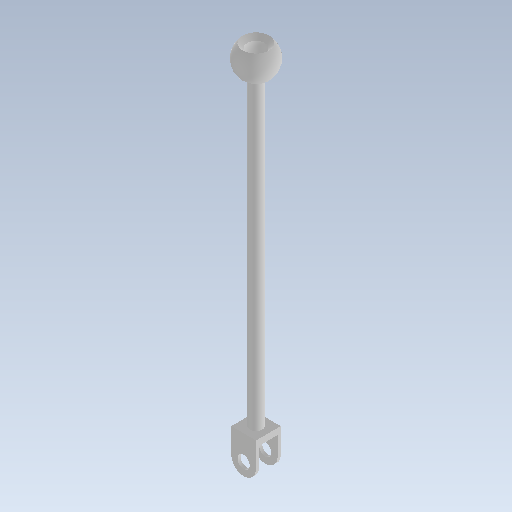
# Autodesk Inventor part: US_Dyad-01
Saved by Autodesk Inventor 2020.1 (Build 241239000, 239)
## iProperties
Created: 2019-10-24
Part Number: US_Dyad-01
Material: Generic
Document SubType Name: Modeling
Designer: sshel
Density: 1 g/cm^3
Appearance: Default
Author: sshel
Autodesk Inventor part; units mm, degrees
ref_plane "YZ Plane" through (0, 0, 0) normal (1, 0, 0) x (0, 1, 0)
ref_plane "XZ Plane" through (0, 0, 0) normal (0, 1, 0) x (-1, 0, 0)
ref_plane "XY Plane" through (0, 0, 0) normal (0, 0, 1) x (1, 0, 0)
sketch "Sketch1" plane through (0, 0, 0) normal (0, 1, 0) x (-1, 0, 0)
  line L0 (0, 0) -> (0, -5145.9)
  line L1 (-200, -4980.2146) -> (-200, 0)
  line L2 (0, 0) -> (-173.6931, 0)
  line L3 (0, 0) -> (0, 5145.9)
  line L4 (-200, 4980.2146) -> (-200, 0)
  arc A0 (-424.2641, 5970.1641) -> (-200, 4980.2146) centre (0, 5545.9) ccw
  arc A1 (-282.8427, 5828.7427) -> (0, 5145.9) centre (0, 5545.9) ccw
  line L5 (-282.8427, 5828.7427) -> (-424.2641, 5970.1641)
  line L6 (0, -7806.6864) -> (0, 8018.8184) construction
  line L7 (0, -5145.9) -> (0, -5545.9)
  line L8 (0, -5545.9) -> (-200, -5545.9)
  line L9 (-200, -5545.9) -> (-200, -4980.2146)
  point P0 (0, -2.2081)
  point P1 (-13.1062, 0)
  point P2 (-20, -18.7767)
  point P3 (-20, 3.1509)
  point P4 (-46.6023, 0)
  point P5 (-20, -18.7767)
  dimension "d6" = 45
  dimension "d7" = 200
  dimension "d8" = 400
  dimension "d9" = 200
  dimension "d10" = 11091.8
  constraints: 18 end point, 4 point on circle, 3 symmetric about line, 2 centre point, 2 horizontal, 2 point on line, 2 vertical, 1 coincident, 1 collinear, 1 perpendicular
  measures "d6" angle of L6 L5
  measures "d7" radial gap between concentric circles of A1 A0
  measures "d8" radius of A1
  measures "d9" distance between parallel lines of L4 L6
  measures "d10" distance of L7.end A1.centre
revolve "Revolution1" add sketch "Sketch1" angle 360 about axis through (0, 0, -10) along (0, 0, 1)
sketch "Sketch2" plane through (0, 0, 0) normal (0, 1, 0) x (-1, 0, 0)
  line L0 (200, -5545.9) -> (-200, -5545.9) projected
  arc A0 (-400, -5545.9) -> (400, -5545.9) centre (0, -5545.9) ccw
  line L1 (65.0556, -5545.9) -> (-85.3956, -5545.9)
  line L2 (0, -338.7665) -> (0, -580.5318)
  line L3 (400, -5545.9) -> (400, -4745.9)
  line L4 (400, -4745.9) -> (-400, -4745.9)
  line L5 (-400, -4745.9) -> (-400, -5545.9)
  point P0 (0, 0)
  dimension "d11" = 400
  dimension "d12" = 800
  constraints: 10 end point, 4 point on line, 2 perpendicular, 2 point on circle, 2 vertical, 1 centre point, 1 horizontal, 1 midpoint, 1 tangent
  measures "d11" radius of A0
  measures "d12" distance of L5.end L4.end
extrude "Extrusion1" add sketch "Sketch2" along normal mid plane 800
sketch "Sketch4" plane through (0, 0, 0) normal (0, 1, 0) x (-1, 0, 0)
  arc A0 (-400, -5545.9) -> (400, -5545.9) centre (0, -5545.9) ccw construction
  circle A1 centre (0, -5545.9) radius 200
  point P0 (0, 0)
  dimension "d16" = 200
  constraints: 1 centre point, 1 coincident
  measures "d16" radius of A1
extrude "Extrusion2" cut sketch "Sketch4" along normal through all both and the other way through all
sketch "Sketch6" plane through (0, 0, 0) normal (1, 0, 0) x (0, 1, 0)
  line L0 (-400, -5945.9) -> (400, -5945.9) construction
  line L1 (0, -623.7458) -> (0, -465.1617)
  line L2 (300, -5945.9) -> (-300, -5945.9)
  line L3 (-300, -5945.9) -> (-300, -4945.9)
  line L4 (-300, -4945.9) -> (300, -4945.9)
  line L5 (300, -4945.9) -> (300, -5945.9)
  point P0 (0, 0)
  point P1 (0, -5945.9)
  dimension "d27" = 600
  dimension "d28" = 1000
  constraints: 10 end point, 2 parallel, 1 collinear, 1 horizontal, 1 midpoint, 1 perpendicular, 1 point on line, 1 vertical, 1 other
  measures "d27" distance between parallel lines of L3 L5
  measures "d28" distance of L2.end L3.end
extrude "Extrusion4" cut sketch "Sketch6" along normal through all both and the other way through all
equation "\"d7\" = rod_radius"
equation "\"d8\" = S_radius"
equation "\"d9\" = rod_radius"
equation "\"d10\" = L1"
equation "\"d11\" = S_radius"
equation "\"d12\" = 2 * S_radius"
equation "\"d13\" = 2 * S_radius"
equation "\"d16\" = rod_radius"
equation "\"d27\" = 3 * rod_radius"
equation "\"d28\" = 5 * rod_radius"
equation "\"L1\" = 11091.8"
equation "\"rod_radius\" = 200"
equation "\"S_radius\" = 2 * rod_radius"
equation "\"dyad1_Fx\" = 500.274"
equation "\"dyad1_Fy\" = -9043.2"
equation "\"dyad1_Fz\" = 3698.67"
equation "\"dyad2_Fx\" = -4998.92"
equation "\"dyad2_Fy\" = 784.414"
equation "\"dyad2_Fz\" = -922.893"
equation "\"dyad3_Fx\" = -9966.37"
equation "\"dyad3_Fy\" = -12953.9"
equation "\"dyad3_Fz\" = 14045.1"
equation "\"dyad4_Fx\" = 15757.5"
equation "\"dyad4_Fy\" = -714.453"
equation "\"dyad4_Fz\" = 4795.98"
equation "\"dyad5_Fx\" = 3128.85"
equation "\"dyad5_Fy\" = -7023.29"
equation "\"dyad5_Fz\" = 14568"
equation "\"L2\" = 11990.4"
equation "\"L3\" = 15457.3"
equation "\"L4\" = 18860.2"
equation "\"L5\" = 20834.9"
body "Solid1"
